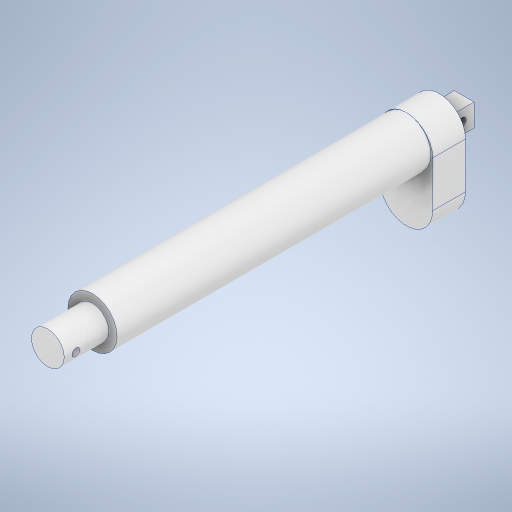
# Autodesk Inventor part: 높이조절 액추에이터_최대
Saved by Autodesk Inventor 2024 (Build 280153000, 153)
## iProperties
Created: 2024-04-09
Part Number: 높이조절 액추에이터_최대
Material: 알루미늄 6061
Document SubType Name: Modeling
Designer: kkamin5
Density: 2.7 g/cm^3
Appearance: 알루미늄 - 평지
Author: kkamin5
Autodesk Inventor part; units mm, degrees
ref_plane "YZ Plane" through (0, 0, 0) normal (1, 0, 0) x (0, 1, 0)
ref_plane "XZ Plane" through (0, 0, 0) normal (0, 1, 0) x (-1, 0, 0)
ref_plane "XY Plane" through (0, 0, 0) normal (0, 0, 1) x (1, 0, 0)
sketch "스케치1" plane through (0, 0, 0) normal (0, 0, 1) x (1, 0, 0)
  line L0 (0, 17.4) -> (0, -17.4) construction
  line L1 (-20, 17.4) -> (-20, -17.4)
  line L2 (20, -17.4) -> (20, 17.4)
  arc A0 (20, 17.4) -> (-20, 17.4) centre (0, 17.4) ccw
  arc A1 (-20, -17.4) -> (20, -17.4) centre (0, -17.4) ccw
  point P0 (0, 0)
  point P1 (0, 0)
  dimension "d0" = 34.8
  dimension "d1" = 40
  constraints: 8 end point, 4 point on circle, 4 tangent, 2 centre point, 1 midpoint, 1 parallel, 1 vertical
  measures "d0" distance of L0.start L0.end
  measures "d1" diameter of A1
extrude "돌출1" add sketch "스케치1" along normal blind 25
sketch "스케치2" plane through (0, 0, 25) normal (0, 0, 1) x (1, 0, 0)
  circle A0 centre (0, 18.7) radius 18.7
  point P0 (0, 0)
  dimension "d4" = 37.4
  constraints: 1 vertical alignment, 2 other
extrude "돌출2" add sketch "스케치2" along normal blind 239
sketch "스케치3" plane through (0, 18.7, 264) normal (0, 0, 1) x (1, 0, 0)
  circle A0 centre (0, 0) radius 12.5
  point P0 (0, -18.7)
  dimension "d7" = 25
  constraints: 1 centre point
  measures "d7" diameter of A0
extrude "돌출3" add sketch "스케치3" along normal blind 34
sketch "스케치5" plane through (0, 0, 0) normal (0, 0, -1) x (-1, 0, 0)
  line L0 (-7.5, 8.75) -> (7.5, 8.75)
  line L1 (7.5, 8.75) -> (7.5, 26.05)
  line L2 (7.5, 26.05) -> (-7.5, 26.05)
  line L3 (-7.5, 26.05) -> (-7.5, 8.75)
  arc A0 (20, 17.4) -> (-20, 17.4) centre (0, 17.4) ccw projected
  point P0 (0, 0)
  dimension "d10" = 15
  dimension "d11" = 17.3
  dimension "d12" = 8.65
  dimension "d13" = 7.5
  constraints: 8 end point, 2 parallel, 1 horizontal, 1 perpendicular
  measures "d10" distance of L2.end L1.end
  measures "d11" distance of L1.end L0.end
  measures "d12" distance from line of A0.centre L2
  measures "d13" distance from line of A0.centre L1
extrude "돌출4" add sketch "스케치5" along normal blind 19
sketch "스케치6" plane through (-20, -17.4, 0) normal (-1, 0, 0) x (0, 0, 1)
  circle A0 centre (-10, 34.8) radius 3
  line L0 (-19, 26.15) -> (-19, 43.45) projected
  line L1 (0, 43.45) -> (-19, 43.45) projected
  circle A1 centre (289, 34.8) radius 3
  line L2 (0, 0) -> (25, 0) projected
  point P0 (0, 17.4)
  dimension "d16" = 6
  dimension "d17" = 9
  dimension "d18" = 8.65
  dimension "d19" = 299
  dimension "d20" = 34.8
  dimension "d21" = 6
  constraints: 2 centre point
  measures "d16" diameter of A0
  measures "d17" distance from line of L0 A0.centre
  measures "d18" distance from line of L1 A0.centre
  measures "d19" distance of A0.centre A1.centre
  measures "d20" distance from line of L2 A1.centre
  measures "d21" diameter of A1
extrude "돌출5" cut sketch "스케치6" against normal through all
